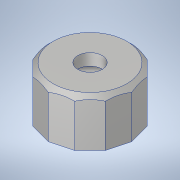
# Autodesk Inventor part: Cubierta
Saved by Autodesk Inventor 2020.2 (Build 242310000, 310)
## iProperties
Created: 2019-09-21
Part Number: Cubierta
Material: Aluminio 6061
Document SubType Name: Modeling
Designer: axelj
Density: 2.7 g/cm^3
Appearance: Aluminio - Plano
Author: axelj
Autodesk Inventor part; units mm, degrees
ref_plane "YZ Plane" through (0, 0, 0) normal (1, 0, 0) x (0, 1, 0)
ref_plane "XZ Plane" through (0, 0, 0) normal (0, 1, 0) x (-1, 0, 0)
ref_plane "XY Plane" through (0, 0, 0) normal (0, 0, 1) x (1, 0, 0)
sketch "Boceto1" plane through (0, 0, 0) normal (0, 1, 0) x (-1, 0, 0)
  circle A0 centre (0, 0) radius 1.45
  dimension "d3" = 2.9
  constraints: 1 centre point, 1 coincident
  measures "d3" diameter of A0
extrude "Extrusión1" add sketch "Boceto1" along normal blind 25
sketch "Boceto3" plane through (0, 0, 0) normal (0, -1, 0) x (1, 0, 0)
  circle A0 centre (0, 0) radius 5
  dimension "d5" = 10
  constraints: 1 centre point, 1 coincident
  measures "d5" diameter of A0
extrude "Extrusión2" add sketch "Boceto3" along normal blind 5.7
chamfer "Chaflán1" distance 0.6 angle 45 1 edges at (-5, 0, 0)
sketch "Boceto5" plane through (0, -5.7, 0) normal (0, -1, 0) x (1, 0, 0)
  line L0 (0, 0) -> (0, 5) construction
  line L1 (0, 0) -> (5, 0) construction
  line L2 (0, 0) -> (4.3301, -2.5) construction
  line L3 (0, 0) -> (5, 0) construction
  line L4 (0, 0) -> (2.5, -4.3301) construction
  line L5 (0, 0) -> (5, 0) construction
  line L6 (0, 0) -> (0, -5) construction
  line L7 (0, 0) -> (5, 0) construction
  line L8 (0, 0) -> (-5, 0) construction
  line L9 (0, 0) -> (-5, 0) construction
  line L10 (0, 0) -> (-4.3301, -2.5) construction
  line L11 (0, 0) -> (-2.5, -4.3301) construction
  line L12 (0, 0) -> (4.3301, 2.5) construction
  line L13 (0, 0) -> (2.5, 4.3301) construction
  line L14 (0, 0) -> (-4.3301, 2.5) construction
  line L15 (0, 0) -> (-2.5, 4.3301) construction
  line L16 (4.3301, -2.5) -> (2.5, -4.3301)
  line L17 (2.5, -4.3301) -> (0, -5)
  line L18 (0, -5) -> (-2.5, -4.3301)
  line L19 (-2.5, -4.3301) -> (-4.3301, -2.5)
  line L20 (-5, 0) -> (-4.3301, 2.5)
  line L21 (-4.3301, 2.5) -> (-2.5, 4.3301)
  line L22 (-2.5, 4.3301) -> (0, 5)
  line L23 (0, 5) -> (2.5, 4.3301)
  line L24 (2.5, 4.3301) -> (4.3301, 2.5)
  line L25 (4.3301, 2.5) -> (5, 0)
  line L26 (5, 0) -> (4.3301, -2.5)
  line L27 (-4.3301, -2.5) -> (-5, 0)
  circle A0 centre (0, 0) radius 5
  dimension "d13" = 5
  dimension "d14" = 30
  dimension "d16" = 60
  constraints: 56 end point, 7 symmetric about line, 6 perpendicular, 4 equal length, 3 horizontal, 1 coincident, 1 point on line, 1 vertical, 1 vertical alignment, 2 other
  measures "d13" distance of L1.start L2.end
  measures "d14" angle of L2 L3
  measures "d16" angle of L4 L5
extrude "Extrusión3" cut sketch "Boceto5" against normal blind 6 contours A0 L16 | L26 A0 | A0 L17 | L25 A0 | A0 L18 | L24 A0 | A0 L19 | L23 A0 | A0 L27 | L22 A0 | A0 L20 | L21 A0
sketch "Boceto7" plane through (0, 25, 0) normal (0, 1, 0) x (1, 0, 0)
  circle A0 centre (0, 0) radius 1.45
  dimension "d22" = 2.9
  constraints: 1 centre point, 1 coincident
  measures "d22" diameter of A0
extrude "Extrusión5" cut sketch "Boceto7" against normal blind 29
sketch "Boceto8" plane through (0, -5.7, 0) normal (0, -1, 0) x (1, 0, 0)
  circle A0 centre (0, 0) radius 4.65
  dimension "d25" = 9.3
  constraints: 1 centre point, 1 coincident
  measures "d25" diameter of A0
extrude "Extrusión6" cut sketch "Boceto8" against normal blind 4.3
thread "Rosca2" size "M9x1.25" class "6H" standard "ANSI Metric M Profile" full length
